Baseplate_v9 (Autodesk Fusion 360 design; units mm, degrees)
Autodesk Fusion 360 part; units mm, degrees
sketch "Sketch1" plane through (0, 0, 0) normal (0, 0, 1) x (1, 0, 0)
  line L0 (239.5, 110) -> (-19.5, 110)
  circle A0 centre (230, 100) radius 2.75
  circle A1 centre (-10, 100) radius 2.75
  line L1 (240, -109.5) -> (240, 109.5)
  circle A2 centre (87, 100) radius 2.75
  circle A3 centre (41, 100) radius 2.75
  line L2 (-20, 109.5) -> (-20, -109.5)
  circle A4 centre (179, 100) radius 2.75
  circle A5 centre (133, 100) radius 2.75
  circle A6 centre (87, -100) radius 2.75
  circle A7 centre (-10, 40) radius 2.75
  circle A8 centre (10, 80) radius 2.75
  circle A9 centre (230, 40) radius 2.75
  circle A10 centre (230, -20) radius 2.75
  circle A11 centre (-10, -40) radius 2.75
  circle A12 centre (230, 20) radius 2.75
  circle A13 centre (-10, -100) radius 2.75
  circle A14 centre (230, -40) radius 2.75
  line L3 (-19.5, -110) -> (239.5, -110)
  circle A15 centre (-10, -20) radius 2.75
  circle A16 centre (41, -100) radius 2.75
  circle A17 centre (-10, 20) radius 2.75
  circle A18 centre (133, -100) radius 2.75
  circle A19 centre (179, -100) radius 2.75
  circle A20 centre (230, -100) radius 2.75
  line L4 (240, 109.5) -> (240, 109.5) construction
  arc A21 (240, 109.5) -> (239.5, 110) centre (239.5, 109.5) ccw
  arc A22 (239.5, -110) -> (240, -109.5) centre (239.5, -109.5) ccw
  arc A23 (-20, -109.5) -> (-19.5, -110) centre (-19.5, -109.5) ccw
  arc A24 (-19.5, 110) -> (-20, 109.5) centre (-19.5, 109.5) ccw
  circle A25 centre (10, 60) radius 2.75
  circle A26 centre (83, 0) radius 2.75
  dimension "d20" = 5.5
  dimension "d21" = 5.5
  dimension "d22" = 5.5
  dimension "d23" = 5.5
  dimension "d24" = 5.5
  dimension "d25" = 5.5
  dimension "d26" = 5.5
  dimension "d27" = 5.5
  dimension "d28" = 5.5
  dimension "d29" = 5.5
  dimension "d30" = 5.5
  dimension "d31" = 5.5
  dimension "d36" = 5.5
  dimension "d43" = 5.5
  dimension "d44" = 5.5
  dimension "d45" = 5.5
  dimension "d46" = 5.5
  dimension "d49" = 5.5
  dimension "d50" = 5.5
  dimension "d51" = 5.5
  dimension "d52" = 5.5
  dimension "d54" = 5.5
  dimension "d56" = 5.5
  constraint horizontal L3
  constraint vertical L1
  constraint horizontal L0
  constraint vertical L2
  measures "d20" diameter of A13
  measures "d21" diameter of A11
  measures "d22" diameter of A15
  measures "d23" diameter of A17
  measures "d24" diameter of A7
  measures "d25" diameter of A1
  measures "d26" diameter of A20
  measures "d27" diameter of A14
  measures "d28" diameter of A10
  measures "d29" diameter of A12
  measures "d30" diameter of A9
  measures "d31" diameter of A0
  measures "d36" diameter of A8
  measures "d43" diameter of A3
  measures "d44" diameter of A2
  measures "d45" diameter of A5
  measures "d46" diameter of A4
  measures "d49" diameter of A16
  measures "d50" diameter of A6
  measures "d51" diameter of A18
  measures "d52" diameter of A19
  measures "d54" diameter of A25
  measures "d56" diameter of A26
extrude "Extrude1" add sketch "Sketch1" along normal blind 3
